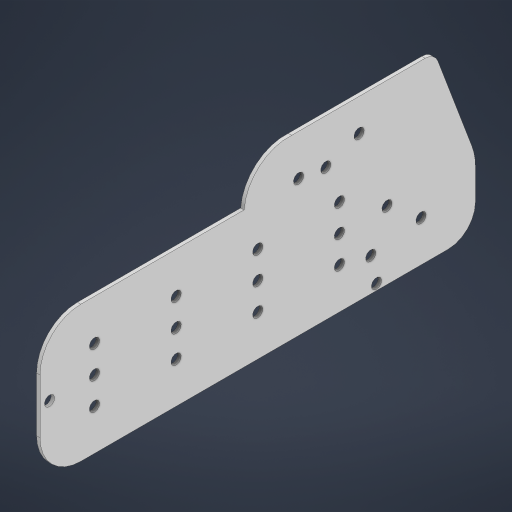
# Autodesk Inventor part: dtplate
Saved by Autodesk Inventor 2024 (Build 280153000, 153)
## iProperties
Created: 2023-11-04
Part Number: dtplate
Material: Generic
Document SubType Name: Modeling
Designer: macbook
Density: 1 g/cm^3
Appearance: Default
Author: macbook
Autodesk Inventor part; units mm, degrees
ref_plane "YZ Plane" through (0, 0, 0) normal (1, 0, 0) x (0, 1, 0)
ref_plane "XZ Plane" through (0, 0, 0) normal (0, 1, 0) x (-1, 0, 0)
ref_plane "XY Plane" through (0, 0, 0) normal (0, 0, 1) x (1, 0, 0)
sketch "Sketch1" plane through (0, 0, 0) normal (1, 0, 0) x (0, 1, 0)
  line L0 (0, -19.05) -> (0, -190.5)
  line L1 (12.7, -203.2) -> (27.1441, -203.2)
  line L2 (63.5, -203.2) -> (63.5, -19.05) construction
  line L3 (0, -25.4) -> (19.05, -25.4) construction
  line L4 (19.05, -25.4) -> (19.05, -63.5) construction
  line L5 (19.05, -63.5) -> (19.05, -101.6) construction
  line L6 (19.05, -101.6) -> (19.05, -139.7) construction
  line L7 (19.05, -25.4) -> (31.75, -25.4) construction
  line L8 (31.75, -25.4) -> (44.45, -25.4) construction
  line L9 (44.45, -25.4) -> (44.45, -63.5) construction
  line L10 (44.45, -63.5) -> (44.45, -101.6) construction
  line L11 (44.45, -101.6) -> (44.45, -139.7) construction
  line L12 (31.75, -25.4) -> (31.75, -63.5) construction
  line L13 (31.75, -63.5) -> (31.75, -101.6) construction
  line L14 (31.75, -101.6) -> (31.75, -139.7) construction
  line L15 (31.75, -139.7) -> (31.75, -161.925) construction
  line L16 (44.45, 0) -> (19.05, 0)
  arc A0 (19.05, 0) -> (0, -19.05) centre (19.05, -19.05) ccw
  arc A1 (63.5, -19.05) -> (44.45, 0) centre (44.45, -19.05) ccw
  line L17 (31.75, -161.925) -> (67.5523, -148.894) construction
  line L18 (31.75, -161.925) -> (69.85, -161.925) construction
  line L19 (19.05, -139.7) -> (19.05, -177.8) construction
  line L20 (31.75, -161.925) -> (19.8159, -166.2687) construction
  line L21 (31.75, -161.925) -> (44.45, -161.925) construction
  line L22 (19.8159, -166.2687) -> (15.4722, -154.3346) construction
  line L23 (15.4722, -154.3346) -> (3.5382, -158.6782) construction
  line L24 (3.5382, -158.6782) -> (2.93, -157.0074)
  line L25 (44.45, -101.6) -> (44.45, -120.65)
  line L26 (44.45, -120.65) -> (63.5, -120.65)
  line L27 (63.5, -120.65) -> (63.5, -133.35)
  line L28 (63.5, -133.35) -> (61.722, -133.35)
  line L29 (63.5, -19.05) -> (63.5, -95.25)
  line L30 (63.5, -203.2) -> (82.55, -203.2)
  line L31 (82.55, -203.2) -> (82.55, -184.15)
  line L32 (63.5, -95.25) -> (63.5, -117.475)
  line L33 (63.5, -117.475) -> (82.55, -117.475) construction
  arc A2 (82.55, -117.475) -> (63.5, -95.25) centre (61.8713, -115.9228) ccw
  line L34 (82.55, -117.475) -> (82.55, -179.7494)
  line L35 (82.55, -203.2) -> (31.75, -203.2)
  line L36 (36.0626, -201.5828) -> (78.4296, -185.6951)
  arc A3 (0, -190.5) -> (12.7, -203.2) centre (12.7, -190.5) ccw
  arc A4 (78.4296, -185.6951) -> (82.55, -179.7494) centre (76.2, -179.7494) ccw
  arc A5 (27.1441, -203.2) -> (36.0626, -201.5828) centre (27.1441, -177.8) ccw
  line L37 (31.75, -25.4) -> (31.75, -4.445) construction
  point P0 (0, 0)
  point P1 (0, -203.2)
  point P2 (63.5, 0)
  point P3 (63.5, -134.85)
  point P4 (63.5, -181.028)
  point P5 (63.5, -191.2938)
  dimension "d0" = 203.2
  dimension "d1" = 63.5
  dimension "d13" = 38.1
  dimension "d14" = 38.1
  dimension "d15" = 38.1
  dimension "d17" = 12.7
  dimension "d18" = 12.7
  dimension "d19" = 22.225
  dimension "d28" = 19.05
  dimension "d29" = 19.05
  dimension "d31" = 38.1
  dimension "d32" = 20
  dimension "d33" = 38.1
  dimension "d34" = 38.1
  dimension "d35" = 38.1
  dimension "d36" = 38.1
  dimension "d40" = 12.7
  dimension "d41" = 160
  dimension "d42" = 12.7
  dimension "d43" = 12.7
  dimension "d44" = 1.778
  dimension "d45" = 19.05
  dimension "d46" = 19.05
  dimension "d48" = 12.7
  dimension "d49" = 1.778
  dimension "d50" = 76.2
  dimension "d51" = 19.05
  dimension "d52" = 19.05
  dimension "d53" = 22.225
  dimension "d54" = 50.8
  dimension "d55" = 12.7
  dimension "d56" = 6.35
  dimension "d57" = 25.4
  dimension "d58" = 20.955
  constraints: 76 end point, 24 point on line, 20 coincident, 12 point on circle, 10 tangent, 7 vertical, 6 centre point, 6 horizontal, 6 perpendicular, 2 equal length, 1 midpoint
  measures "d0" distance of point (0, 0) point (0, -203.2)
  measures "d1" distance of point (0, 0) point (63.5, 0)
  measures "d13" distance of L4.start L4.end
  measures "d14" distance of L4.end L5.end
  measures "d15" distance of L5.end L6.end
  measures "d17" distance of L4.start L7.end
  measures "d18" distance of L7.end L8.end
  measures "d19" distance of L15.start L15.end
  measures "d28" radius of A0
  measures "d29" radius of A1
  measures "d31" distance of L17.start L17.end
  measures "d32" angle of L18 L17
  measures "d33" distance of L19.start L19.end
  measures "d34" distance of L13.end L14.end
  measures "d35" distance of L12.end L13.end
  measures "d36" distance of L7.end L12.end
  measures "d40" distance of L17.start L20.end
  measures "d41" angle of L20 L21
  measures "d42" distance of L20.end L22.end
  measures "d43" distance of L23.start L23.end
  measures "d44" distance of L23.end L24.end
  measures "d45" distance of L25.start L25.end
  measures "d46" distance of L25.end L26.end
  measures "d48" distance of L27.start L27.end
  measures "d49" distance of L27.end L28.end
  measures "d50" distance of L2.end L29.end
  measures "d51" distance of L2.start L30.end
  measures "d52" distance of L30.end L31.end
  measures "d53" distance of L29.end L32.end
  measures "d54" distance of L30.end L35.end
  measures "d55" radius of A3
  measures "d56" radius of A4
  measures "d57" radius of A5
  measures "d58" distance of L37.start L37.end
extrude "Extrusion1" add sketch "Sketch1" along normal blind 1.5875
hole "Hole2" at (0, 19.05, -25.4) at (0, 19.05, -63.5) at (0, 19.05, -101.6) at (0, 19.05, -139.7) at (0, 44.45, -25.4) at (0, 31.75, -25.4) at (0, 31.75, -63.5) at (0, 44.45, -63.5) at (0, 31.75, -101.6) at (0, 44.45, -101.6) at (0, 31.75, -139.7) at (0, 44.45, -139.7) at (0, 31.75, -161.925) at (0, 67.5523, -148.894) at (0, 19.05, -177.8) at (0, 15.4722, -154.3346) at (0, 2.93, -157.0074) at (0, 63.5, -120.65) at (0, 61.722, -133.35) at (0, 31.75, -4.445) direction (1, 0, 0) diameter 4.7625 end through all
body "Solid1"
